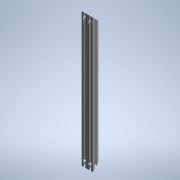
# Autodesk Inventor part: 20-2568_b
Saved by Autodesk Inventor 2021 (Build 250183000, 183)
## iProperties
Part Number: 20-2568_b
Material: Generic
Catalog Web Link: www.cadenas.de
Description: 20-2566, 20-2567, 20-2568, 20-2566-Black, 20-2567-Black, 20-2568-Black_b-20 Series - T-Slotted Profile
Vendor: 8020
Document SubType Name: Modeling
Designer: partserver
Manufacturer: 8020
Mass: 123.727 g
Surface Area: 1499.82 cm^2
Volume: 123.727 cm^3
Density: 1 g/cm^3
Appearance: PSOLRGB-191-191-191
Category: PARTsolutions
Company: 8020
PSOL_IDENT_0: {$CADENAS_DATA\23d-libs\8020\metric\joining_plates\20_2040_m.prj},231 {VTYP=3D},{NB=20-2568_b},{LINA=
PSOL_IDENT_1: 20-2568},{NN=20-2566, 20-2567, 20-2568, 20-2566-Black, 20-2567-Black, 20-2568-Black_b},{DATE=31.07.2
PSOL_IDENT_2: 020 09:21:28},{GEOMDATE=21.12.2017 20:05:16},{VERSION=},{LINEID=10},{WBVAR=FINISH,L},{WBNUMERIC=L}
PSOL_IDENT_3: {NB=20-2568_b},{LINA=20-2568},{KT=DUMMY},{PN=20-2568},{FINISH=CA},{L=480.00},{SERIES=20-2040-M},{MAT=
PSOL_IDENT_4: 6105-T5 Aluminum},{W=.7426},{LALG=160,320,480},{MIX=1.215},{MIY=4.546},{EA=2.75},{CLR=.75,.75,.75}
NB: 20-2568_b
NN: 20-2566, 20-2567, 20-2568, 20-2566-Black, 20-2567-Black, 20-2568-Black_b
NT: 20 Series - T-Slotted Profile
NBSYN: $PN._b
LINA: 20-2568
CATALOG: 80/20
PN: 20-2568
FINISH: Clear Anodize
L: 480
MAT: 6105-T5 Aluminum
W: .7426
MIX: 1.215
MIY: 4.546
EA: 2.75
SUPPLIER: 8020
ARTICLENO: 20-2568_b
BOMINFO: 20-2568
CREATOR: CADENAS GmbH
Title: 20-2568
Author: Cadenas PARTsolutions
Comments: 20 Series - T-Slotted Profile
Autodesk Inventor part; units mm, degrees
sketch "Sketch_1" plane through (0, 0, 0) normal (0, 0, 1) x (1, 0, 0)
  arc A0 (-20, -8.5014) -> (-18.5014, -10) centre (-18.5014, -8.5014) ccw
  line L0 (-18.5014, -10) -> (-17.2568, -10)
  line L1 (-17.2568, -10) -> (-13.1192, -9.8555)
  arc A1 (-13.1192, -9.8555) -> (-12.6293, -9.3285) centre (-13.1369, -9.3478) ccw
  line L2 (-12.6293, -9.3285) -> (-12.6476, -8.8462)
  arc A2 (-12.6476, -8.8462) -> (-13.173, -8.3579) centre (-13.1553, -8.8656) ccw
  line L3 (-13.173, -8.3579) -> (-15.4687, -8.438)
  arc A3 (-15.9944, -7.9304) -> (-15.4687, -8.438) centre (-15.4864, -7.9304) ccw
  line L4 (-15.9944, -7.9304) -> (-15.9944, -7.2645)
  arc A4 (-15.8456, -6.9053) -> (-15.9944, -7.2645) centre (-15.4864, -7.2645) ccw
  line L5 (-15.8456, -6.9053) -> (-12.7477, -3.8074)
  arc A5 (-12.3885, -3.6586) -> (-12.7477, -3.8074) centre (-12.3885, -4.1666) ccw
  line L6 (-12.3885, -3.6586) -> (-7.6115, -3.6586)
  arc A6 (-7.2523, -3.8074) -> (-7.6115, -3.6586) centre (-7.6115, -4.1666) ccw
  line L7 (-7.2523, -3.8074) -> (-4.1544, -6.9053)
  arc A7 (-4.0056, -7.2645) -> (-4.1544, -6.9053) centre (-4.5136, -7.2645) ccw
  line L8 (-4.0056, -7.2645) -> (-4.0056, -7.9304)
  arc A8 (-4.5313, -8.438) -> (-4.0056, -7.9304) centre (-4.5136, -7.9304) ccw
  line L9 (-4.5313, -8.438) -> (-6.827, -8.3579)
  arc A9 (-6.827, -8.3579) -> (-7.3524, -8.8462) centre (-6.8447, -8.8656) ccw
  line L10 (-7.3524, -8.8462) -> (-7.3707, -9.3285)
  arc A10 (-7.3707, -9.3285) -> (-6.8808, -9.8555) centre (-6.8631, -9.3478) ccw
  line L11 (-6.8808, -9.8555) -> (-2.7432, -10)
  line L12 (-2.7432, -10) -> (2.7432, -10)
  line L13 (2.7432, -10) -> (6.8808, -9.8555)
  arc A11 (6.8808, -9.8555) -> (7.3707, -9.3285) centre (6.8631, -9.3478) ccw
  line L14 (7.3707, -9.3285) -> (7.3524, -8.8462)
  arc A12 (7.3524, -8.8462) -> (6.827, -8.3579) centre (6.8447, -8.8656) ccw
  line L15 (6.827, -8.3579) -> (4.5313, -8.438)
  arc A13 (4.0056, -7.9304) -> (4.5313, -8.438) centre (4.5136, -7.9304) ccw
  line L16 (4.0056, -7.9304) -> (4.0056, -7.2645)
  arc A14 (4.1544, -6.9053) -> (4.0056, -7.2645) centre (4.5136, -7.2645) ccw
  line L17 (4.1544, -6.9053) -> (7.2523, -3.8074)
  arc A15 (7.6115, -3.6586) -> (7.2523, -3.8074) centre (7.6115, -4.1666) ccw
  line L18 (7.6115, -3.6586) -> (12.3885, -3.6586)
  arc A16 (12.7477, -3.8074) -> (12.3885, -3.6586) centre (12.3885, -4.1666) ccw
  line L19 (12.7477, -3.8074) -> (15.8456, -6.9053)
  arc A17 (15.9944, -7.2645) -> (15.8456, -6.9053) centre (15.4864, -7.2645) ccw
  line L20 (15.9944, -7.2645) -> (15.9944, -7.9304)
  arc A18 (15.4687, -8.438) -> (15.9944, -7.9304) centre (15.4864, -7.9304) ccw
  line L21 (15.4687, -8.438) -> (13.173, -8.3579)
  arc A19 (13.173, -8.3579) -> (12.6476, -8.8462) centre (13.1553, -8.8656) ccw
  line L22 (12.6476, -8.8462) -> (12.6293, -9.3285)
  arc A20 (12.6293, -9.3285) -> (13.1192, -9.8555) centre (13.1369, -9.3478) ccw
  line L23 (13.1192, -9.8555) -> (17.2568, -10)
  line L24 (17.2568, -10) -> (18.5014, -10)
  arc A21 (18.5014, -10) -> (20, -8.5014) centre (18.5014, -8.5014) ccw
  line L25 (20, -8.5014) -> (20, -7.2568)
  line L26 (20, -7.2568) -> (19.8555, -3.1192)
  arc A22 (19.8555, -3.1192) -> (19.3285, -2.6293) centre (19.3478, -3.1369) ccw
  line L27 (19.3285, -2.6293) -> (18.8462, -2.6476)
  arc A23 (18.8462, -2.6476) -> (18.3579, -3.173) centre (18.8656, -3.1553) ccw
  line L28 (18.3579, -3.173) -> (18.438, -5.4687)
  arc A24 (17.9304, -5.9944) -> (18.438, -5.4687) centre (17.9304, -5.4864) ccw
  line L29 (17.9304, -5.9944) -> (17.2645, -5.9944)
  arc A25 (16.9053, -5.8456) -> (17.2645, -5.9944) centre (17.2645, -5.4864) ccw
  line L30 (16.9053, -5.8456) -> (13.8074, -2.7477)
  arc A26 (13.6586, -2.3885) -> (13.8074, -2.7477) centre (14.1666, -2.3885) ccw
  line L31 (13.6586, -2.3885) -> (13.6586, 2.3885)
  arc A27 (13.8074, 2.7477) -> (13.6586, 2.3885) centre (14.1666, 2.3885) ccw
  line L32 (13.8074, 2.7477) -> (16.9053, 5.8456)
  arc A28 (17.2645, 5.9944) -> (16.9053, 5.8456) centre (17.2645, 5.4864) ccw
  line L33 (17.2645, 5.9944) -> (17.9304, 5.9944)
  arc A29 (18.438, 5.4687) -> (17.9304, 5.9944) centre (17.9304, 5.4864) ccw
  line L34 (18.438, 5.4687) -> (18.3579, 3.173)
  arc A30 (18.3579, 3.173) -> (18.8462, 2.6476) centre (18.8656, 3.1553) ccw
  line L35 (18.8462, 2.6476) -> (19.3285, 2.6293)
  arc A31 (19.3285, 2.6293) -> (19.8555, 3.1192) centre (19.3478, 3.1369) ccw
  line L36 (19.8555, 3.1192) -> (20, 7.2568)
  line L37 (20, 7.2568) -> (20, 8.5014)
  arc A32 (20, 8.5014) -> (18.5014, 10) centre (18.5014, 8.5014) ccw
  line L38 (18.5014, 10) -> (17.2568, 10)
  line L39 (17.2568, 10) -> (13.1192, 9.8555)
  arc A33 (13.1192, 9.8555) -> (12.6293, 9.3285) centre (13.1369, 9.3478) ccw
  line L40 (12.6293, 9.3285) -> (12.6476, 8.8462)
  arc A34 (12.6476, 8.8462) -> (13.173, 8.3579) centre (13.1553, 8.8656) ccw
  line L41 (13.173, 8.3579) -> (15.4687, 8.438)
  arc A35 (15.9944, 7.9304) -> (15.4687, 8.438) centre (15.4864, 7.9304) ccw
  line L42 (15.9944, 7.9304) -> (15.9944, 7.2645)
  arc A36 (15.8456, 6.9053) -> (15.9944, 7.2645) centre (15.4864, 7.2645) ccw
  line L43 (15.8456, 6.9053) -> (12.7477, 3.8074)
  arc A37 (12.3885, 3.6586) -> (12.7477, 3.8074) centre (12.3885, 4.1666) ccw
  line L44 (12.3885, 3.6586) -> (7.6115, 3.6586)
  arc A38 (7.2523, 3.8074) -> (7.6115, 3.6586) centre (7.6115, 4.1666) ccw
  line L45 (7.2523, 3.8074) -> (4.1544, 6.9053)
  arc A39 (4.0056, 7.2645) -> (4.1544, 6.9053) centre (4.5136, 7.2645) ccw
  line L46 (4.0056, 7.2645) -> (4.0056, 7.9304)
  arc A40 (4.5313, 8.438) -> (4.0056, 7.9304) centre (4.5136, 7.9304) ccw
  line L47 (4.5313, 8.438) -> (6.827, 8.3579)
  arc A41 (6.827, 8.3579) -> (7.3524, 8.8462) centre (6.8447, 8.8656) ccw
  line L48 (7.3524, 8.8462) -> (7.3707, 9.3285)
  arc A42 (7.3707, 9.3285) -> (6.8808, 9.8555) centre (6.8631, 9.3478) ccw
  line L49 (6.8808, 9.8555) -> (2.7432, 10)
  line L50 (2.7432, 10) -> (-2.7432, 10)
  line L51 (-2.7432, 10) -> (-6.8808, 9.8555)
  arc A43 (-6.8808, 9.8555) -> (-7.3707, 9.3285) centre (-6.8631, 9.3478) ccw
  line L52 (-7.3707, 9.3285) -> (-7.3524, 8.8462)
  arc A44 (-7.3524, 8.8462) -> (-6.827, 8.3579) centre (-6.8447, 8.8656) ccw
  line L53 (-6.827, 8.3579) -> (-4.5313, 8.438)
  arc A45 (-4.0056, 7.9304) -> (-4.5313, 8.438) centre (-4.5136, 7.9304) ccw
  line L54 (-4.0056, 7.9304) -> (-4.0056, 7.2645)
  arc A46 (-4.1544, 6.9053) -> (-4.0056, 7.2645) centre (-4.5136, 7.2645) ccw
  line L55 (-4.1544, 6.9053) -> (-7.2523, 3.8074)
  arc A47 (-7.6115, 3.6586) -> (-7.2523, 3.8074) centre (-7.6115, 4.1666) ccw
  line L56 (-7.6115, 3.6586) -> (-12.3885, 3.6586)
  arc A48 (-12.7477, 3.8074) -> (-12.3885, 3.6586) centre (-12.3885, 4.1666) ccw
  line L57 (-12.7477, 3.8074) -> (-15.8456, 6.9053)
  arc A49 (-15.9944, 7.2645) -> (-15.8456, 6.9053) centre (-15.4864, 7.2645) ccw
  line L58 (-15.9944, 7.2645) -> (-15.9944, 7.9304)
  arc A50 (-15.4687, 8.438) -> (-15.9944, 7.9304) centre (-15.4864, 7.9304) ccw
  line L59 (-15.4687, 8.438) -> (-13.173, 8.3579)
  arc A51 (-13.173, 8.3579) -> (-12.6476, 8.8462) centre (-13.1553, 8.8656) ccw
  line L60 (-12.6476, 8.8462) -> (-12.6293, 9.3285)
  arc A52 (-12.6293, 9.3285) -> (-13.1192, 9.8555) centre (-13.1369, 9.3478) ccw
  line L61 (-13.1192, 9.8555) -> (-17.2568, 10)
  line L62 (-17.2568, 10) -> (-18.5014, 10)
  arc A53 (-18.5014, 10) -> (-20, 8.5014) centre (-18.5014, 8.5014) ccw
  line L63 (-20, 8.5014) -> (-20, 7.2568)
  line L64 (-20, 7.2568) -> (-19.8555, 3.1192)
  arc A54 (-19.8555, 3.1192) -> (-19.3285, 2.6293) centre (-19.3478, 3.1369) ccw
  line L65 (-19.3285, 2.6293) -> (-18.8462, 2.6476)
  arc A55 (-18.8462, 2.6476) -> (-18.3579, 3.173) centre (-18.8656, 3.1553) ccw
  line L66 (-18.3579, 3.173) -> (-18.438, 5.4687)
  arc A56 (-17.9304, 5.9944) -> (-18.438, 5.4687) centre (-17.9304, 5.4864) ccw
  line L67 (-17.9304, 5.9944) -> (-17.2645, 5.9944)
  arc A57 (-16.9053, 5.8456) -> (-17.2645, 5.9944) centre (-17.2645, 5.4864) ccw
  line L68 (-16.9053, 5.8456) -> (-13.8074, 2.7477)
  arc A58 (-13.6586, 2.3885) -> (-13.8074, 2.7477) centre (-14.1666, 2.3885) ccw
  line L69 (-13.6586, 2.3885) -> (-13.6586, -2.3885)
  arc A59 (-13.8074, -2.7477) -> (-13.6586, -2.3885) centre (-14.1666, -2.3885) ccw
  line L70 (-13.8074, -2.7477) -> (-16.9053, -5.8456)
  arc A60 (-17.2645, -5.9944) -> (-16.9053, -5.8456) centre (-17.2645, -5.4864) ccw
  line L71 (-17.2645, -5.9944) -> (-17.9304, -5.9944)
  arc A61 (-18.438, -5.4687) -> (-17.9304, -5.9944) centre (-17.9304, -5.4864) ccw
  line L72 (-18.438, -5.4687) -> (-18.3579, -3.173)
  arc A62 (-18.3579, -3.173) -> (-18.8462, -2.6476) centre (-18.8656, -3.1553) ccw
  line L73 (-18.8462, -2.6476) -> (-19.3285, -2.6293)
  arc A63 (-19.3285, -2.6293) -> (-19.8555, -3.1192) centre (-19.3478, -3.1369) ccw
  line L74 (-19.8555, -3.1192) -> (-20, -7.2568)
  line L75 (-20, -7.2568) -> (-20, -8.5014)
  arc A64 (7.8707, -0.8806) -> (7.7034, -2.1217) centre (8.2602, -1.565) ccw
  line L76 (7.7034, -2.1217) -> (7.8783, -2.2966)
  arc A65 (7.8783, -2.2966) -> (9.1194, -2.1293) centre (8.435, -1.7398) ccw
  arc A66 (9.4115, -2.0112) -> (9.1194, -2.1293) centre (9.3401, -2.2549) ccw
  arc A67 (9.4115, -2.0112) -> (10.5885, -2.0112) centre (10, 0) ccw
  arc A68 (10.8806, -2.1293) -> (10.5885, -2.0112) centre (10.6599, -2.2549) ccw
  arc A69 (10.8806, -2.1293) -> (12.1217, -2.2966) centre (11.565, -1.7398) ccw
  line L77 (12.1217, -2.2966) -> (12.2966, -2.1217)
  arc A70 (12.2966, -2.1217) -> (12.1293, -0.8806) centre (11.7398, -1.565) ccw
  arc A71 (12.0112, -0.5885) -> (12.1293, -0.8806) centre (12.2549, -0.6599) ccw
  arc A72 (12.0112, -0.5885) -> (12.0112, 0.5885) centre (10, 0) ccw
  arc A73 (12.1293, 0.8806) -> (12.0112, 0.5885) centre (12.2549, 0.6599) ccw
  arc A74 (12.1293, 0.8806) -> (12.2966, 2.1217) centre (11.7398, 1.565) ccw
  line L78 (12.2966, 2.1217) -> (12.1217, 2.2966)
  arc A75 (12.1217, 2.2966) -> (10.8806, 2.1293) centre (11.565, 1.7398) ccw
  arc A76 (10.5885, 2.0112) -> (10.8806, 2.1293) centre (10.6599, 2.2549) ccw
  arc A77 (10.5885, 2.0112) -> (9.4115, 2.0112) centre (10, 0) ccw
  arc A78 (9.1194, 2.1293) -> (9.4115, 2.0112) centre (9.3401, 2.2549) ccw
  arc A79 (9.1194, 2.1293) -> (7.8783, 2.2966) centre (8.435, 1.7398) ccw
  line L79 (7.8783, 2.2966) -> (7.7034, 2.1217)
  arc A80 (7.7034, 2.1217) -> (7.8707, 0.8806) centre (8.2602, 1.565) ccw
  arc A81 (7.9888, 0.5885) -> (7.8707, 0.8806) centre (7.7451, 0.6599) ccw
  arc A82 (7.9888, 0.5885) -> (7.9888, -0.5885) centre (10, 0) ccw
  arc A83 (7.8707, -0.8806) -> (7.9888, -0.5885) centre (7.7451, -0.6599) ccw
  line L80 (-6.3414, 2.3885) -> (-6.3414, -2.3885)
  arc A84 (-6.3414, -2.3885) -> (-6.1926, -2.7477) centre (-5.8334, -2.3885) ccw
  line L81 (-6.1926, -2.7477) -> (-2.6558, -6.2845)
  arc A85 (-2.507, -6.6438) -> (-2.6558, -6.2845) centre (-3.015, -6.6438) ccw
  line L82 (-2.507, -6.6438) -> (-2.507, -7.9934)
  arc A86 (-2.507, -7.9934) -> (-1.999, -8.5014) centre (-1.999, -7.9934) ccw
  line L83 (-1.999, -8.5014) -> (1.999, -8.5014)
  arc A87 (1.999, -8.5014) -> (2.507, -7.9934) centre (1.999, -7.9934) ccw
  line L84 (2.507, -7.9934) -> (2.507, -6.6438)
  arc A88 (2.6558, -6.2845) -> (2.507, -6.6438) centre (3.015, -6.6438) ccw
  line L85 (2.6558, -6.2845) -> (6.1926, -2.7477)
  arc A89 (6.1926, -2.7477) -> (6.3414, -2.3885) centre (5.8334, -2.3885) ccw
  line L86 (6.3414, -2.3885) -> (6.3414, 2.3885)
  arc A90 (6.3414, 2.3885) -> (6.1926, 2.7477) centre (5.8334, 2.3885) ccw
  line L87 (6.1926, 2.7477) -> (2.6558, 6.2845)
  arc A91 (2.507, 6.6438) -> (2.6558, 6.2845) centre (3.015, 6.6438) ccw
  line L88 (2.507, 6.6438) -> (2.507, 7.9934)
  arc A92 (2.507, 7.9934) -> (1.999, 8.5014) centre (1.999, 7.9934) ccw
  line L89 (1.999, 8.5014) -> (-1.999, 8.5014)
  arc A93 (-1.999, 8.5014) -> (-2.507, 7.9934) centre (-1.999, 7.9934) ccw
  line L90 (-2.507, 7.9934) -> (-2.507, 6.6438)
  arc A94 (-2.6558, 6.2845) -> (-2.507, 6.6438) centre (-3.015, 6.6438) ccw
  line L91 (-2.6558, 6.2845) -> (-6.1926, 2.7477)
  arc A95 (-6.1926, 2.7477) -> (-6.3414, 2.3885) centre (-5.8334, 2.3885) ccw
  arc A96 (-12.2966, 2.1217) -> (-12.1293, 0.8806) centre (-11.7398, 1.565) ccw
  arc A97 (-12.0112, 0.5885) -> (-12.1293, 0.8806) centre (-12.2549, 0.6599) ccw
  arc A98 (-12.0112, 0.5885) -> (-12.0112, -0.5885) centre (-10, 0) ccw
  arc A99 (-12.1293, -0.8806) -> (-12.0112, -0.5885) centre (-12.2549, -0.6599) ccw
  arc A100 (-12.1293, -0.8806) -> (-12.2966, -2.1217) centre (-11.7398, -1.565) ccw
  line L92 (-12.2966, -2.1217) -> (-12.1217, -2.2966)
  arc A101 (-12.1217, -2.2966) -> (-10.8806, -2.1293) centre (-11.565, -1.7398) ccw
  arc A102 (-10.5885, -2.0112) -> (-10.8806, -2.1293) centre (-10.6599, -2.2549) ccw
  arc A103 (-10.5885, -2.0112) -> (-9.4115, -2.0112) centre (-10, 0) ccw
  arc A104 (-9.1194, -2.1293) -> (-9.4115, -2.0112) centre (-9.3401, -2.2549) ccw
  arc A105 (-9.1194, -2.1293) -> (-7.8783, -2.2966) centre (-8.435, -1.7398) ccw
  line L93 (-7.8783, -2.2966) -> (-7.7034, -2.1217)
  arc A106 (-7.7034, -2.1217) -> (-7.8707, -0.8806) centre (-8.2602, -1.565) ccw
  arc A107 (-7.9888, -0.5885) -> (-7.8707, -0.8806) centre (-7.7451, -0.6599) ccw
  arc A108 (-7.9888, -0.5885) -> (-7.9888, 0.5885) centre (-10, 0) ccw
  arc A109 (-7.8707, 0.8806) -> (-7.9888, 0.5885) centre (-7.7451, 0.6599) ccw
  arc A110 (-7.8707, 0.8806) -> (-7.7034, 2.1217) centre (-8.2602, 1.565) ccw
  line L94 (-7.7034, 2.1217) -> (-7.8783, 2.2966)
  arc A111 (-7.8783, 2.2966) -> (-9.1194, 2.1293) centre (-8.435, 1.7398) ccw
  arc A112 (-9.4115, 2.0112) -> (-9.1194, 2.1293) centre (-9.3401, 2.2549) ccw
  arc A113 (-9.4115, 2.0112) -> (-10.5885, 2.0112) centre (-10, 0) ccw
  arc A114 (-10.8806, 2.1293) -> (-10.5885, 2.0112) centre (-10.6599, 2.2549) ccw
  arc A115 (-10.8806, 2.1293) -> (-12.1217, 2.2966) centre (-11.565, 1.7398) ccw
  line L95 (-12.1217, 2.2966) -> (-12.2966, 2.1217)
  constraints: 232 point on circle, 192 end point, 116 centre point
extrude "Extrusion1" add sketch "Sketch_1" along normal mid plane 480
sketch "Sketch_2" plane through (0, 0, 0) normal (1, 0, 0) x (0, 1, 0)
  line L0 (17.5, 245) -> (-12.5, 245)
  line L1 (-12.5, 245) -> (-12.5, 240)
  line L2 (-12.5, 240) -> (12.5, 215)
  line L3 (12.5, 215) -> (12.5, -215)
  line L4 (12.5, -215) -> (-12.5, -240)
  line L5 (-12.5, -240) -> (-12.5, -245)
  line L6 (-12.5, -245) -> (17.5, -245)
  line L7 (17.5, -245) -> (17.5, 245)
  constraints: 16 end point
extrude "Extrusion2" cut sketch "Sketch_2" along normal mid plane 50
sketch "Sketch_3" plane through (10, 0, 0) normal (1, 0, 0) x (0, 0, -1)
  line L0 (-209.8223, -17.6777) -> (-227.5, 0)
  line L1 (-227.5, 0) -> (-225.6262, 1.8738)
  line L2 (-225.6262, 1.8738) -> (-222.0906, -1.6617)
  line L3 (-222.0906, -1.6617) -> (-219.4743, 0.9546)
  line L4 (-219.4743, 0.9546) -> (-205.3322, -13.1875)
  line L5 (-205.3322, -13.1875) -> (-209.8223, -17.6777)
  line L6 (-209.8223, -17.6777) -> (-227.5, 0)
  constraints: 14 end point
revolve "Revolution1" cut sketch "Sketch_3" angle 360 about axis through (10, -17.6777, 209.8223) along (0, -0.7071, -0.7071)
sketch "Sketch_4" plane through (10, 0, 0) normal (1, 0, 0) x (0, 0, -1)
  line L0 (227.5, 0) -> (209.8223, -17.6777)
  line L1 (209.8223, -17.6777) -> (205.3322, -13.1875)
  line L2 (205.3322, -13.1875) -> (219.4743, 0.9546)
  line L3 (219.4743, 0.9546) -> (222.0906, -1.6617)
  line L4 (222.0906, -1.6617) -> (225.6262, 1.8738)
  line L5 (225.6262, 1.8738) -> (227.5, 0)
  line L6 (227.5, 0) -> (209.8223, -17.6777)
  constraints: 14 end point
revolve "Revolution2" cut sketch "Sketch_4" angle 360 about axis through (10, 0, -227.5) along (0, 0.7071, -0.7071)
sketch "Sketch_5" plane through (-10, 0, 0) normal (1, 0, 0) x (0, 0, -1)
  line L0 (-209.8223, -17.6777) -> (-227.5, 0)
  line L1 (-227.5, 0) -> (-225.6262, 1.8738)
  line L2 (-225.6262, 1.8738) -> (-222.0906, -1.6617)
  line L3 (-222.0906, -1.6617) -> (-219.4743, 0.9546)
  line L4 (-219.4743, 0.9546) -> (-205.3322, -13.1875)
  line L5 (-205.3322, -13.1875) -> (-209.8223, -17.6777)
  line L6 (-209.8223, -17.6777) -> (-227.5, 0)
  constraints: 14 end point
revolve "Revolution3" cut sketch "Sketch_5" angle 360 about axis through (-10, -17.6777, 209.8223) along (0, -0.7071, -0.7071)
sketch "Sketch_6" plane through (-10, 0, 0) normal (1, 0, 0) x (0, 0, -1)
  line L0 (227.5, 0) -> (209.8223, -17.6777)
  line L1 (209.8223, -17.6777) -> (205.3322, -13.1875)
  line L2 (205.3322, -13.1875) -> (219.4743, 0.9546)
  line L3 (219.4743, 0.9546) -> (222.0906, -1.6617)
  line L4 (222.0906, -1.6617) -> (225.6262, 1.8738)
  line L5 (225.6262, 1.8738) -> (227.5, 0)
  line L6 (227.5, 0) -> (209.8223, -17.6777)
  constraints: 14 end point
revolve "Revolution4" cut sketch "Sketch_6" angle 360 about axis through (-10, 0, -227.5) along (0, 0.7071, -0.7071)
ref_plane "1_XY" through (10, -3.5355, 223.9645) normal (0, 0.7071, 0.7071) x (1, 0, 0)
ref_plane "1_YZ" through (10, -3.5355, 223.9645) normal (1, 0, 0) x (0, 0.7071, -0.7071)
ref_plane "1_ZX" through (10, -3.5355, 223.9645) normal (0, 0.7071, -0.7071) x (0, 0.7071, 0.7071)
ref_plane "2_XY" through (-10, -3.5355, 223.9645) normal (0, 0.7071, 0.7071) x (1, 0, 0)
ref_plane "2_YZ" through (-10, -3.5355, 223.9645) normal (1, 0, 0) x (0, 0.7071, -0.7071)
ref_plane "2_ZX" through (-10, -3.5355, 223.9645) normal (0, 0.7071, -0.7071) x (0, 0.7071, 0.7071)
ref_plane "3_XY" through (10, -3.5355, -223.9645) normal (0, -0.7071, 0.7071) x (1, 0, 0)
ref_plane "3_YZ" through (10, -3.5355, -223.9645) normal (1, 0, 0) x (0, 0.7071, 0.7071)
ref_plane "3_ZX" through (10, -3.5355, -223.9645) normal (0, 0.7071, 0.7071) x (0, -0.7071, 0.7071)
ref_plane "4_XY" through (-10, -3.5355, -223.9645) normal (0, -0.7071, 0.7071) x (1, 0, 0)
ref_plane "4_YZ" through (-10, -3.5355, -223.9645) normal (1, 0, 0) x (0, 0.7071, 0.7071)
ref_plane "4_ZX" through (-10, -3.5355, -223.9645) normal (0, 0.7071, 0.7071) x (0, -0.7071, 0.7071)
ref_plane "to_dummy_XY" through (0, 0, 0) normal (0, 1, 0) x (1, 0, 0)
ref_plane "to_dummy_YZ" through (0, 0, 0) normal (1, 0, 0) x (0, 0, -1)
ref_plane "to_dummy_ZX" through (0, 0, 0) normal (0, 0, -1) x (0, 1, 0)
body "Solid1"
